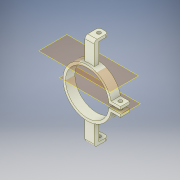
# Autodesk Inventor part: SupportBracket_v2_BilgePumpMotor
Saved by Autodesk Inventor 2019 (Build 230136000, 136)
## iProperties
Created: 2019-03-02
Part Number: SupportBracket_v2_BilgePumpMotor
Material: ABS Plastic
Document SubType Name: Modeling
Designer: User
Density: 1.06 g/cm^3
Appearance: Smooth - Ivory
Author: User
Autodesk Inventor part; units mm, degrees
ref_plane "XY Plane" through (0, 0, 0) normal (0, 0, 1) x (1, 0, 0)
sketch "Sketch1" plane through (0, 0, 0) normal (0, 0, 1) x (1, 0, 0)
  arc A0 (23.1619, 2.0217) -> (23.1619, -2.0217) centre (0, 0) ccw
  arc A1 (25.5104, 5.0217) -> (25.5104, -5.0217) centre (0, 0) ccw
  line L0 (23.1619, 2.0217) -> (35.5104, 2.0217)
  line L1 (25.5104, 5.0217) -> (35.5104, 5.0217)
  line L2 (35.5104, 5.0217) -> (35.5104, 2.0217)
  line L3 (0, 0) -> (18.0567, 0)
  line L4 (23.1619, -2.0217) -> (35.5104, -2.0217)
  line L5 (25.5104, -5.0217) -> (35.5104, -5.0217)
  line L6 (35.5104, -5.0217) -> (35.5104, -2.0217)
  dimension "d0" = 46.5
  dimension "d1" = 52
  dimension "d33" = 3
  dimension "d34" = 10
  constraints: 14 end point, 4 point on circle, 3 symmetric about line, 2 centre point, 2 coincident, 2 horizontal, 1 parallel, 1 perpendicular
  measures "d0" diameter of A0
  measures "d1" diameter of A1
  measures "d33" distance between parallel lines of L0 L1
  measures "d34" distance of L1.start L1.end
extrude "Extrusion1" add sketch "Sketch1" against normal blind 10
sketch "Sketch2" plane through (24.6779, 5.0217, 0) normal (0, 1, 0) x (1, 0, 0)
  line L0 (10.8325, 0) -> (0.8325, 0) projected
  line L1 (10.8325, 0) -> (10.8325, 10) projected
  line L2 (0.8325, 10) -> (10.8325, 10) projected
  line L3 (0.8325, 0) -> (0.8325, 10) projected
  circle A0 centre (5.8325, 5) radius 2
  point P0 (-24.6779, 0)
  dimension "d35" = 4
  constraints: 1 centre point
  measures "d35" diameter of A0
extrude "Extrusion2" cut sketch "Sketch2" against normal blind 11 contours A0
ref_plane "Work Plane3" through (24.6779, 24, 0) normal (0, 1, 0) x (1, 0, 0)
sketch "Sketch3" plane through (24.6779, 24, 0) normal (0, 1, 0) x (1, 0, 0)
  line L0 (-24.6779, 0) -> (-24.6779, 10)
  line L1 (-19.6779, 7.5) -> (-29.6779, 7.5)
  line L2 (-29.6779, 2.5) -> (-19.6779, 2.5)
  line L3 (-19.6779, 2.5) -> (-19.6779, 7.5)
  line L4 (-29.6779, 2.5) -> (-29.6779, 7.5)
  point P0 (-24.6779, 5)
  constraints: 10 end point, 1 coincident, 1 midpoint, 1 parallel, 1 vertical
extrude "Extrusion3" add sketch "Sketch3" along normal blind 22.5
ref_plane "Work Plane4" through (5, 25.5147, -6) normal (1, 0, 0) x (0, 0, -1)
sketch "Sketch4" plane through (5, 25.5147, -6) normal (1, 0, 0) x (0, 0, -1)
  line L0 (-3.5, 20.9853) -> (1.5, 20.9853) projected
  line L1 (-3.5, 20.9853) -> (11.5, 20.9853)
  line L2 (11.5, 20.9853) -> (11.5, 23.9853)
  line L3 (11.5, 23.9853) -> (-3.5, 23.9853)
  line L4 (-3.5, 23.9853) -> (-3.5, 20.9853)
  point P0 (-6, -24.4949)
  dimension "d36" = 15
  dimension "d37" = 3
  constraints: 8 end point, 2 parallel, 1 horizontal, 1 perpendicular
  measures "d36" distance of L3.end L2.end
  measures "d37" distance of L2.end L1.end
extrude "Extrusion4" add sketch "Sketch4" against normal blind 10
ref_plane "Work Plane2" through (0, 0, 0) normal (0.7071068, -0.7071068, 0) x (0, 0, -1)
sketch "Sketch5" plane through (5, 49.5, -2.5) normal (0, 1, 0) x (1, 0, 0)
  circle A0 centre (-5, 10) radius 2
  dimension "d29" = 4
  constraints: 1 centre point
  measures "d29" diameter of A0
extrude "Extrusion5" cut sketch "Sketch5" against normal blind 4
fillet "Fillet2" radius 3 3 edges at (0, 49.5, -2.5) (5, 48, -17.5) (-5, 48, -17.5)
mirror "Mirror3" about plane through (0, 0, 0) normal (0, 1, 0) of "Extrusion4", "Fillet2", "Extrusion3", "Extrusion5"
body "Solid1"
